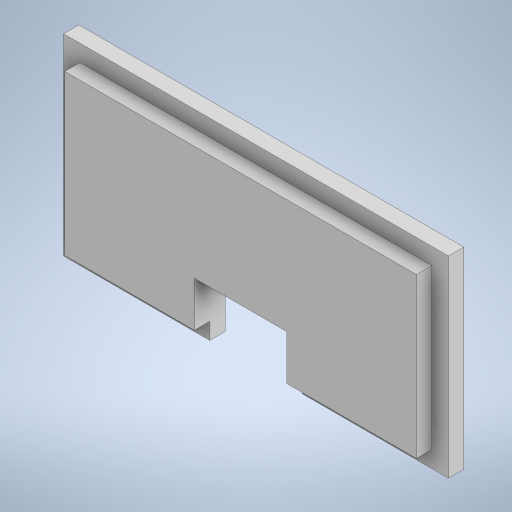
# Autodesk Inventor part: UltrasonicSensorMountTest_backplate
Saved by Autodesk Inventor 2024.2 (Build 282272000, 272)
## iProperties
Created: 2024-04-02
Part Number: UltrasonicSensorMountTest_backplate
Material: Generic
Document SubType Name: Modeling
Designer: ringl
Density: 1 g/cm^3
Appearance: Default
Author: ringl
Autodesk Inventor part; units mm, degrees
ref_plane "YZ Plane" through (0, 0, 0) normal (1, 0, 0) x (0, 1, 0)
ref_plane "XZ Plane" through (0, 0, 0) normal (0, 1, 0) x (-1, 0, 0)
ref_plane "XY Plane" through (0, 0, 0) normal (0, 0, 1) x (1, 0, 0)
sketch "Sketch1" plane through (0, 0, 0) normal (0, 0, 1) x (1, 0, 0)
  line L0 (0, 0) -> (50, 0)
  line L1 (50, 0) -> (50, -25)
  line L2 (50, -25) -> (0, -25)
  line L3 (0, -25) -> (0, 0)
  dimension "d0" = 50
  dimension "d1" = 25
  constraints: 8 end point, 2 parallel, 1 coincident, 1 horizontal, 1 perpendicular
  measures "d0" distance of L1.end L2.end
  measures "d1" distance of L0.end L1.end
extrude "Extrusion1" add sketch "Sketch1" along normal blind 2
sketch "Sketch2" plane through (0, 0, 2) normal (0, 0, 1) x (1, 0, 0)
  line L0 (47.85, -2.15) -> (2.15, -2.15)
  line L1 (2.15, -2.15) -> (2.15, -22.85)
  line L2 (2.15, -22.85) -> (47.85, -22.85)
  line L3 (47.85, -22.85) -> (47.85, -2.15)
  line L4 (50, -25) -> (50, 0) projected
  line L5 (50, 0) -> (0, 0) projected
  dimension "d4" = 45.7
  dimension "d5" = 20.7
  dimension "d6" = 2.15
  dimension "d7" = 2.15
  constraints: 8 end point, 2 parallel, 1 horizontal, 1 perpendicular
  measures "d4" distance of L2.end L1.end
  measures "d5" distance of L1.end L0.end
  measures "d6" distance between parallel lines of L3 L4
  measures "d7" distance between parallel lines of L5 L0
extrude "Extrusion2" add sketch "Sketch2" along normal blind 2
sketch "Sketch3" plane through (0, 0, 0) normal (0, 0, -1) x (-1, 0, 0)
  line L0 (0, -25) -> (-50, -25) projected
  line L1 (-19, -25) -> (-31, -25)
  line L2 (-31, -25) -> (-31, -17)
  line L3 (-31, -17) -> (-19, -17)
  line L4 (-19, -17) -> (-19, -25)
  line L5 (0, 0) -> (0, -25) projected
  dimension "d10" = 12
  dimension "d11" = 8
  dimension "d12" = 19
  constraints: 8 end point, 2 parallel, 1 horizontal, 1 perpendicular, 1 point on line
  measures "d10" distance of L2.end L3.end
  measures "d11" distance of L1.end L2.end
  measures "d12" distance between parallel lines of L5 L4
extrude "Extrusion3" cut sketch "Sketch3" against normal through all
body "Solid1"
